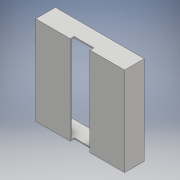
# Autodesk Inventor part: weight_holder
Saved by Autodesk Inventor 2017 (Build 210142000, 142)
## iProperties
Created: 2016-06-06
Part Number: weight_holder
Material: Generic
Document SubType Name: Modeling
Designer: Conor
Density: 1 g/cm^3
Appearance: Default
Author: Conor
Autodesk Inventor part; units mm, degrees
ref_plane "YZ Plane" through (0, 0, 0) normal (1, 0, 0) x (0, 1, 0)
ref_plane "XZ Plane" through (0, 0, 0) normal (0, 1, 0) x (-1, 0, 0)
ref_plane "XY Plane" through (0, 0, 0) normal (0, 0, 1) x (1, 0, 0)
sketch "Sketch1" plane through (0, 0, 0) normal (0, 1, 0) x (-1, 0, 0)
  line L0 (28.1728, 44.1076) -> (-61.8272, 44.1076)
  line L1 (-61.8272, 44.1076) -> (-61.8272, -45.8924)
  line L2 (-61.8272, -45.8924) -> (28.1728, -45.8924)
  line L3 (28.1728, -45.8924) -> (28.1728, 44.1076)
  point P0 (0, 0)
  dimension "d0" = 90
  dimension "d1" = 90
  constraints: 8 end point, 2 parallel, 1 horizontal, 1 perpendicular
  measures "d0" distance of L2.end L0.start
  measures "d1" distance of L1.end L2.end
extrude "Extrusion1" add sketch "Sketch1" along normal blind 20
sketch "Sketch2" plane through (0, 20, 0) normal (0, 1, 0) x (1, 0, 0)
  line L0 (-26.9728, -42.9076) -> (60.6272, -42.9076)
  line L1 (60.6272, -42.9076) -> (60.6272, 44.6924)
  line L2 (60.6272, 44.6924) -> (-26.9728, 44.6924)
  line L3 (-26.9728, 44.6924) -> (-26.9728, -42.9076)
  line L4 (-28.1728, 45.8924) -> (-28.1728, -44.1076) projected
  line L5 (61.8272, 45.8924) -> (-28.1728, 45.8924) projected
  line L6 (61.8272, -44.1076) -> (61.8272, 45.8924) projected
  line L7 (-28.1728, -44.1076) -> (61.8272, -44.1076) projected
  point P0 (0, 0)
  dimension "d4" = 1.2
  dimension "d5" = 1.2
  dimension "d6" = 1.2
  dimension "d7" = 1.2
  constraints: 8 end point, 2 parallel, 1 horizontal, 1 perpendicular
  measures "d4" distance between parallel lines of L4 L3
  measures "d5" distance between parallel lines of L5 L2
  measures "d6" distance between parallel lines of L6 L1
  measures "d7" distance between parallel lines of L7 L0
extrude "Extrusion2" cut sketch "Sketch2" against normal blind 18.8 contours L3 L2 L1 L0
sketch "Sketch3" plane through (-28.1728, 0, 44.1076) normal (0, 0, 1) x (1, 0, 0)
  line L0 (35, 4) -> (55, 4)
  line L1 (55, 4) -> (55, 0)
  line L2 (55, 0) -> (35, 0)
  line L3 (35, 0) -> (35, 4)
  line L4 (0, 0) -> (90, 0) projected
  line L5 (90, 0) -> (90, 20) projected
  point P0 (28.1728, 0)
  dimension "d10" = 20
  dimension "d11" = 4
  dimension "d12" = 35
  constraints: 8 end point, 2 parallel, 1 collinear, 1 horizontal, 1 perpendicular
  measures "d10" distance of L0.start L0.end
  measures "d11" distance of L0.end L1.end
  measures "d12" distance between parallel lines of L5 L1
extrude "Extrusion3" cut sketch "Sketch3" against normal blind 90
equation "\"d5\" = d4"
equation "\"d6\" = d4"
equation "\"d7\" = d4"
equation "\"d8\" = d2 - d4"
equation "\"d12\" = -0.5 * d10 + 0.5 * d0"
equation "\"d13\" = d0"
equation "\"d2\" = 20"
body "Solid1"
